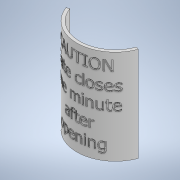
# Autodesk Inventor part: warningSign
Saved by Autodesk Inventor 2021.2 (Build 252289000, 289)
## iProperties
Created: 2020-11-24
Part Number: warningSign
Material: Generic
Document SubType Name: Modeling
Designer: robst
Density: 1 g/cm^3
Appearance: Default
Author: robst
Autodesk Inventor part; units mm, degrees
(part 1 of 2)
ref_plane "YZ Plane" through (0, 0, 0) normal (1, 0, 0) x (0, 1, 0)
ref_plane "XZ Plane" through (0, 0, 0) normal (0, 1, 0) x (-1, 0, 0)
sketch "Sketch1" plane through (0, 0, 0) normal (0, 1, 0) x (-1, 0, 0)
  arc A0 (65.9911, 38.1) -> (-65.4234, 39.0668) centre (0, 0) ccw
  arc A1 (72.6124, 39.2675) -> (-71.4904, 41.275) centre (0, 0) ccw
  line L0 (0, 0) -> (0, -82.55) construction
  arc A2 (71.6046, 26.0619) -> (-71.6046, 26.0619) centre (0, 0) ccw
  arc A3 (77.5716, 28.2338) -> (-77.5716, 28.2338) centre (0, 0) ccw
  line L1 (0, 0) -> (77.5716, 28.2338) construction
  line L2 (0, 0) -> (-77.5716, 28.2338) construction
  line L3 (-77.5716, 28.2338) -> (-71.6046, 26.0619)
  line L4 (77.5716, 28.2338) -> (71.6046, 26.0619)
  point P0 (-65.4234, 39.0668)
  point P1 (65.9911, 38.1)
  point P2 (72.6124, 39.2675)
  point P3 (-71.4904, 41.275)
  dimension "d0" = 152.4
  dimension "d9" = 6.35
  dimension "d10" = 110
  dimension "d11" = 110
  constraints: 10 end point, 8 point on circle, 4 centre point, 4 coincident, 2 concentric, 2 point on line, 1 vertical
  measures "d0" diameter of A0
  measures "d9" radial gap between concentric circles of A1 A0
  measures "d10" angle of L1 L0
  measures "d11" angle of L2 L0
extrude "Extrusion1" add sketch "Sketch1" along normal blind 203.2
ref_plane "Work Plane1" through (0, 0, 82.55) normal (0, 0, 1) x (1, 0, 0)
sketch "Sketch3" plane through (0, 0, 82.55) normal (0, 0, 1) x (1, 0, 0)
  line L0 (-72.043, 0) -> (-72.043, 203.2) projected
  line L1 (71.4904, 0) -> (71.4904, 203.2) projected
  line L2 (77.5716, 203.2) -> (-77.5716, 203.2) projected
  line L3 (77.5716, 0) -> (-77.5716, 0) projected
  line L4 (-72.043, 177.8) -> (71.4904, 177.8) construction
  spline S0 degree 2 poles (-53.3534, 166.2913) (-55.5146, 166.2913) (-59.1708, 167.7501) (-60.5035, 169.209) knots 0 0 0 1 2 2 2
  spline S1 degree 2 poles (-60.5035, 169.209) (-61.8363, 170.6498) (-63.2952, 174.9723) (-63.2952, 177.782) knots 0 0 0 1 2 2 2
  spline S2 degree 2 poles (-63.2952, 177.782) (-63.2952, 180.5736) (-61.8723, 184.716) (-60.5215, 186.2469) knots 0 0 0 1 2 2 2
  spline S3 degree 2 poles (-60.5215, 186.2469) (-59.1888, 187.7418) (-55.5506, 189.3087) (-53.2993, 189.3087) knots 0 0 0 1 2 2 2
  spline S4 degree 2 poles (-53.2993, 189.3087) (-52.1827, 189.3087) (-50.2195, 188.9845) (-49.391, 188.7324) knots 0 0 0 1 2 2 2
  spline S5 degree 2 poles (-49.391, 188.7324) (-48.6706, 188.4983) (-47.1757, 187.8319) (-46.4373, 187.4356) knots 0 0 0 1 2 2 2
  line L5 (-46.4373, 187.4356) -> (-46.4373, 183.8696)
  line L6 (-46.4373, 183.8696) -> (-46.6714, 183.8696)
  spline S6 degree 2 poles (-46.6714, 183.8696) (-47.0677, 184.2298) (-48.2924, 185.2384) (-49.1749, 185.7246) knots 0 0 0 1 2 2 2
  spline S7 degree 2 poles (-49.1749, 185.7246) (-50.0214, 186.1929) (-52.0206, 186.7873) (-53.3173, 186.7873) knots 0 0 0 1 2 2 2
  spline S8 degree 2 poles (-53.3173, 186.7873) (-54.7402, 186.7873) (-57.2796, 185.6166) (-58.2342, 184.4999) knots 0 0 0 1 2 2 2
  spline S9 degree 2 poles (-58.2342, 184.4999) (-59.1708, 183.3653) (-60.2154, 179.9252) (-60.2154, 177.782) knots 0 0 0 1 2 2 2
  spline S10 degree 2 poles (-60.2154, 177.782) (-60.2154, 175.4947) (-59.1167, 172.1987) (-58.1622, 171.0641) knots 0 0 0 1 2 2 2
  spline S11 degree 2 poles (-58.1622, 171.0641) (-57.2256, 169.9654) (-54.7222, 168.8488) (-53.3173, 168.8488) knots 0 0 0 1 2 2 2
  spline S12 degree 2 poles (-53.3173, 168.8488) (-52.0386, 168.8488) (-49.8593, 169.4791) (-49.0128, 169.9474) knots 0 0 0 1 2 2 2
  spline S13 degree 2 poles (-49.0128, 169.9474) (-48.2023, 170.4157) (-46.9956, 171.3882) (-46.6534, 171.7304) knots 0 0 0 1 2 2 2
  line L7 (-46.6534, 171.7304) -> (-46.4373, 171.7304)
  line L8 (-46.4373, 171.7304) -> (-46.4373, 168.2004)
  spline S14 degree 2 poles (-46.4373, 168.2004) (-47.1757, 167.8582) (-48.4725, 167.2278) (-49.391, 166.9396) knots 0 0 0 1 2 2 2
  spline S15 degree 2 poles (-49.391, 166.9396) (-50.3636, 166.6155) (-52.0206, 166.2913) (-53.3534, 166.2913) knots 0 0 0 1 2 2 2
  line L9 (-46.0771, 166.6875) -> (-38.5847, 188.9125)
  line L10 (-38.5847, 188.9125) -> (-34.9466, 188.9125)
  line L11 (-34.9466, 188.9125) -> (-27.4542, 166.6875)
  line L12 (-27.4542, 166.6875) -> (-30.57, 166.6875)
  line L13 (-30.57, 166.6875) -> (-32.5872, 172.9011)
  line L14 (-32.5872, 172.9011) -> (-41.0702, 172.9011)
  line L15 (-41.0702, 172.9011) -> (-43.0873, 166.6875)
  line L16 (-43.0873, 166.6875) -> (-46.0771, 166.6875)
  line L17 (-33.3977, 175.4226) -> (-36.8377, 185.8867)
  line L18 (-36.8377, 185.8867) -> (-40.2597, 175.4226)
  line L19 (-40.2597, 175.4226) -> (-33.3977, 175.4226)
  spline S16 degree 2 poles (-17.2963, 166.2192) (-19.2594, 166.2192) (-22.1771, 167.2458) (-23.2037, 168.2724) knots 0 0 0 1 2 2 2
  spline S17 degree 2 poles (-23.2037, 168.2724) (-24.3744, 169.4251) (-25.329, 172.667) (-25.329, 175.0444) knots 0 0 0 1 2 2 2
  line L20 (-25.329, 175.0444) -> (-25.329, 188.9125)
  line L21 (-25.329, 188.9125) -> (-22.3752, 188.9125)
  line L22 (-22.3752, 188.9125) -> (-22.3752, 175.0444)
  spline S18 degree 2 poles (-22.3752, 175.0444) (-22.3752, 173.4955) (-21.979, 171.4063) (-21.4207, 170.5598) knots 0 0 0 1 2 2 2
  spline S19 degree 2 poles (-21.4207, 170.5598) (-20.8263, 169.6592) (-18.7731, 168.7407) (-17.2963, 168.7407) knots 0 0 0 1 2 2 2
  spline S20 degree 2 poles (-17.2963, 168.7407) (-15.9094, 168.7407) (-13.7482, 169.6592) (-13.1538, 170.5598) knots 0 0 0 1 2 2 2
  spline S21 degree 2 poles (-13.1538, 170.5598) (-12.5955, 171.4063) (-12.1993, 173.4775) (-12.1993, 174.9723) knots 0 0 0 1 2 2 2
  line L23 (-12.1993, 174.9723) -> (-12.1993, 188.9125)
  line L24 (-12.1993, 188.9125) -> (-9.2456, 188.9125)
  line L25 (-9.2456, 188.9125) -> (-9.2456, 175.0444)
  spline S22 degree 2 poles (-9.2456, 175.0444) (-9.2456, 172.721) (-10.1821, 169.4071) (-11.3708, 168.2724) knots 0 0 0 1 2 2 2
  spline S23 degree 2 poles (-11.3708, 168.2724) (-12.4334, 167.2278) (-15.2431, 166.2192) (-17.2963, 166.2192) knots 0 0 0 1 2 2 2
  line L26 (0.174, 166.6875) -> (0.174, 186.283)
  line L27 (0.174, 186.283) -> (-7.2824, 186.283)
  line L28 (-7.2824, 186.283) -> (-7.2824, 188.9125)
  line L29 (-7.2824, 188.9125) -> (10.584, 188.9125)
  line L30 (10.584, 188.9125) -> (10.584, 186.283)
  line L31 (10.584, 186.283) -> (3.1277, 186.283)
  line L32 (3.1277, 186.283) -> (3.1277, 166.6875)
  line L33 (3.1277, 166.6875) -> (0.174, 166.6875)
  line L34 (20.5979, 166.6875) -> (11.9889, 166.6875)
  line L35 (11.9889, 166.6875) -> (11.9889, 168.9568)
  line L36 (11.9889, 168.9568) -> (14.8165, 168.9568)
  line L37 (14.8165, 168.9568) -> (14.8165, 186.6432)
  line L38 (14.8165, 186.6432) -> (11.9889, 186.6432)
  line L39 (11.9889, 186.6432) -> (11.9889, 188.9125)
  line L40 (11.9889, 188.9125) -> (20.5979, 188.9125)
  line L41 (20.5979, 188.9125) -> (20.5979, 186.6432)
  line L42 (20.5979, 186.6432) -> (17.7703, 186.6432)
  line L43 (17.7703, 186.6432) -> (17.7703, 168.9568)
  line L44 (17.7703, 168.9568) -> (20.5979, 168.9568)
  line L45 (20.5979, 168.9568) -> (20.5979, 166.6875)
  spline S24 degree 2 poles (39.9772, 186.373) (41.238, 184.8962) (42.6428, 180.5736) (42.6428, 177.8) knots 0 0 0 1 2 2 2
  spline S25 degree 2 poles (42.6428, 177.8) (42.6428, 175.0984) (41.274, 170.7219) (39.9772, 169.245) knots 0 0 0 1 2 2 2
  spline S26 degree 2 poles (39.9772, 169.245) (38.6084, 167.6961) (34.9883, 166.2192) (32.809, 166.2192) knots 0 0 0 1 2 2 2
  spline S27 degree 2 poles (32.809, 166.2192) (30.5577, 166.2192) (26.9556, 167.7501) (25.6409, 169.245) knots 0 0 0 1 2 2 2
  spline S28 degree 2 poles (25.6409, 169.245) (24.3621, 170.7219) (22.9933, 175.0624) (22.9933, 177.8) knots 0 0 0 1 2 2 2
  spline S29 degree 2 poles (22.9933, 177.8) (22.9933, 180.5916) (24.3801, 184.8421) (25.6589, 186.373) knots 0 0 0 1 2 2 2
  spline S30 degree 2 poles (25.6589, 186.373) (26.9556, 187.8499) (30.5757, 189.3808) (32.809, 189.3808) knots 0 0 0 1 2 2 2
  spline S31 degree 2 poles (32.809, 189.3808) (35.0784, 189.3808) (38.7165, 187.7958) (39.9772, 186.373) knots 0 0 0 1 2 2 2
  spline S32 degree 2 poles (39.563, 177.8) (39.563, 179.9973) (38.6084, 183.4013) (37.7439, 184.5179) knots 0 0 0 1 2 2 2
  spline S33 degree 2 poles (37.7439, 184.5179) (36.8614, 185.6706) (34.376, 186.8233) (32.8271, 186.8233) knots 0 0 0 1 2 2 2
  spline S34 degree 2 poles (32.8271, 186.8233) (31.2241, 186.8233) (28.8107, 185.7066) (27.8922, 184.5179) knots 0 0 0 1 2 2 2
  spline S35 degree 2 poles (27.8922, 184.5179) (27.0097, 183.3833) (26.0731, 179.9613) (26.0731, 177.8) knots 0 0 0 1 2 2 2
  spline S36 degree 2 poles (26.0731, 177.8) (26.0731, 173.4234) (29.7473, 168.7767) (32.8271, 168.7767) knots 0 0 0 1 2 2 2
  spline S37 degree 2 poles (32.8271, 168.7767) (35.9069, 168.7767) (39.563, 173.4234) (39.563, 177.8) knots 0 0 0 1 2 2 2
  line L46 (61.788, 166.6875) -> (58.4741, 166.6875)
  line L47 (58.4741, 166.6875) -> (48.6403, 185.8507)
  line L48 (48.6403, 185.8507) -> (48.6403, 166.6875)
  line L49 (48.6403, 166.6875) -> (45.8847, 166.6875)
  line L50 (45.8847, 166.6875) -> (45.8847, 188.9125)
  line L51 (45.8847, 188.9125) -> (50.0812, 188.9125)
  line L52 (50.0812, 188.9125) -> (59.0324, 171.3162)
  line L53 (59.0324, 171.3162) -> (59.0324, 188.9125)
  line L54 (59.0324, 188.9125) -> (61.788, 188.9125)
  line L55 (61.788, 188.9125) -> (61.788, 166.6875)
  spline S38 degree 2 poles (-65.3844, 129.0315) (-67.7438, 129.0315) (-71.6521, 130.4723) (-73.0569, 131.9312) knots 0 0 0 1 2 2 2
  spline S39 degree 2 poles (-73.0569, 131.9312) (-74.4617, 133.408) (-75.9566, 137.7666) (-75.9566, 140.5942) knots 0 0 0 1 2 2 2
  spline S40 degree 2 poles (-75.9566, 140.5942) (-75.9566, 143.2778) (-74.4437, 147.5283) (-73.0389, 149.0412) knots 0 0 0 1 2 2 2
  spline S41 degree 2 poles (-73.0389, 149.0412) (-71.6881, 150.5) (-67.7258, 152.085) (-65.3664, 152.085) knots 0 0 0 1 2 2 2
  spline S42 degree 2 poles (-65.3664, 152.085) (-64.2317, 152.085) (-62.1785, 151.7608) (-61.242, 151.4726) knots 0 0 0 1 2 2 2
  spline S43 degree 2 poles (-61.242, 151.4726) (-60.4855, 151.2565) (-58.6484, 150.464) (-58.0901, 150.1759) knots 0 0 0 1 2 2 2
  line L56 (-58.0901, 150.1759) -> (-58.0901, 146.6098)
  line L57 (-58.0901, 146.6098) -> (-58.3423, 146.6098)
  spline S44 degree 2 poles (-58.3423, 146.6098) (-58.9006, 147.096) (-60.0713, 147.9786) (-61.1519, 148.4829) knots 0 0 0 1 2 2 2
  spline S45 degree 2 poles (-61.1519, 148.4829) (-62.0524, 148.9331) (-64.3758, 149.5275) (-65.7086, 149.5275) knots 0 0 0 1 2 2 2
  spline S46 degree 2 poles (-65.7086, 149.5275) (-68.9145, 149.5275) (-72.8768, 144.7006) (-72.8768, 140.6843) knots 0 0 0 1 2 2 2
  spline S47 degree 2 poles (-72.8768, 140.6843) (-72.8768, 138.451) (-71.8322, 135.101) (-70.8416, 133.9484) knots 0 0 0 1 2 2 2
  spline S48 degree 2 poles (-70.8416, 133.9484) (-69.887, 132.7957) (-67.1854, 131.589) (-65.4925, 131.589) knots 0 0 0 1 2 2 2
  spline S49 degree 2 poles (-65.4925, 131.589) (-64.2497, 131.589) (-61.7643, 131.9492) (-60.9178, 132.3094) knots 0 0 0 1 2 2 2
  line L58 (-60.9178, 132.3094) -> (-60.9178, 138.0548)
  line L59 (-60.9178, 138.0548) -> (-66.0688, 138.0548)
  line L60 (-66.0688, 138.0548) -> (-66.0688, 140.6483)
  line L61 (-66.0688, 140.6483) -> (-58.0001, 140.6483)
  line L62 (-58.0001, 140.6483) -> (-58.0001, 130.9406)
  spline S50 degree 2 poles (-58.0001, 130.9406) (-58.5584, 130.6885) (-60.4675, 129.914) (-61.278, 129.6799) knots 0 0 0 1 2 2 2
  spline S51 degree 2 poles (-61.278, 129.6799) (-62.3766, 129.3557) (-64.1417, 129.0315) (-65.3844, 129.0315) knots 0 0 0 1 2 2 2
  spline S52 degree 2 poles (-45.2126, 131.2288) (-45.5548, 130.9766) (-46.7075, 130.0761) (-47.2478, 129.8059) knots 0 0 0 1 2 2 2
  spline S53 degree 2 poles (-47.2478, 129.8059) (-47.9862, 129.4097) (-49.373, 128.9955) (-50.6338, 128.9955) knots 0 0 0 1 2 2 2
  spline S54 degree 2 poles (-50.6338, 128.9955) (-51.6604, 128.9955) (-53.5154, 129.7699) (-54.2179, 130.4723) knots 0 0 0 1 2 2 2
  spline S55 degree 2 poles (-54.2179, 130.4723) (-54.8842, 131.1567) (-55.6947, 133.1739) (-55.6947, 134.2906) knots 0 0 0 1 2 2 2
  spline S56 degree 2 poles (-55.6947, 134.2906) (-55.6947, 136.0196) (-54.2359, 138.469) (-52.6509, 139.1714) knots 0 0 0 1 2 2 2
  spline S57 degree 2 poles (-52.6509, 139.1714) (-51.2461, 139.8198) (-47.4279, 140.3061) (-45.2126, 140.4322) knots 0 0 0 1 2 2 2
  line L63 (-45.2126, 140.4322) -> (-45.2126, 140.9725)
  spline S58 degree 2 poles (-45.2126, 140.9725) (-45.2126, 141.945) (-45.8069, 143.1517) (-46.3473, 143.4939) knots 0 0 0 1 2 2 2
  spline S59 degree 2 poles (-46.3473, 143.4939) (-46.8876, 143.8361) (-48.4365, 144.0523) (-49.265, 144.0523) knots 0 0 0 1 2 2 2
  spline S60 degree 2 poles (-49.265, 144.0523) (-50.2375, 144.0523) (-52.8671, 143.4759) (-54.1818, 142.9176) knots 0 0 0 1 2 2 2
  line L64 (-54.1818, 142.9176) -> (-54.3439, 142.9176)
  line L65 (-54.3439, 142.9176) -> (-54.3439, 145.7813)
  spline S61 degree 2 poles (-54.3439, 145.7813) (-53.5695, 145.9974) (-50.6698, 146.5377) (-49.2469, 146.5377) knots 0 0 0 1 2 2 2
  spline S62 degree 2 poles (-49.2469, 146.5377) (-47.5179, 146.5377) (-45.1586, 145.9974) (-44.222, 145.295) knots 0 0 0 1 2 2 2
  spline S63 degree 2 poles (-44.222, 145.295) (-43.3035, 144.6106) (-42.4029, 142.4313) (-42.4029, 140.8644) knots 0 0 0 1 2 2 2
  line L66 (-42.4029, 140.8644) -> (-42.4029, 129.4637)
  line L67 (-42.4029, 129.4637) -> (-45.2126, 129.4637)
  line L68 (-45.2126, 129.4637) -> (-45.2126, 131.2288)
  line L69 (-45.2126, 133.5701) -> (-45.2126, 138.1988)
  spline S64 degree 2 poles (-45.2126, 138.1988) (-46.2212, 138.1088) (-49.265, 137.8026) (-50.2195, 137.5144) knots 0 0 0 1 2 2 2
  spline S65 degree 2 poles (-50.2195, 137.5144) (-51.3362, 137.1722) (-52.795, 135.7494) (-52.795, 134.4887) knots 0 0 0 1 2 2 2
  spline S66 degree 2 poles (-52.795, 134.4887) (-52.795, 133.0478) (-51.1741, 131.589) (-49.6252, 131.589) knots 0 0 0 1 2 2 2
  spline S67 degree 2 poles (-49.6252, 131.589) (-48.3104, 131.589) (-46.1491, 132.7236) (-45.2126, 133.5701) knots 0 0 0 1 2 2 2
  spline S68 degree 2 poles (-33.4157, 129.1395) (-35.703, 129.1395) (-38.2785, 131.7511) (-38.2785, 134.5787) knots 0 0 0 1 2 2 2
  line L70 (-38.2785, 134.5787) -> (-38.2785, 143.8181)
  line L71 (-38.2785, 143.8181) -> (-40.1696, 143.8181)
  line L72 (-40.1696, 143.8181) -> (-40.1696, 146.1415)
  line L73 (-40.1696, 146.1415) -> (-38.2785, 146.1415)
  line L74 (-38.2785, 146.1415) -> (-38.2785, 150.9323)
  line L75 (-38.2785, 150.9323) -> (-35.4689, 150.9323)
  line L76 (-35.4689, 150.9323) -> (-35.4689, 146.1415)
  line L77 (-35.4689, 146.1415) -> (-30.2999, 146.1415)
  line L78 (-30.2999, 146.1415) -> (-30.2999, 143.8181)
  line L79 (-30.2999, 143.8181) -> (-35.4689, 143.8181)
  line L80 (-35.4689, 143.8181) -> (-35.4689, 135.8755)
  spline S69 degree 2 poles (-35.4689, 135.8755) (-35.4689, 134.6147) (-35.3788, 133.2279) (-35.0727, 132.6336) knots 0 0 0 1 2 2 2
  spline S70 degree 2 poles (-35.0727, 132.6336) (-34.8205, 132.1113) (-33.6858, 131.589) (-32.7133, 131.589) knots 0 0 0 1 2 2 2
  spline S71 degree 2 poles (-32.7133, 131.589) (-32.0289, 131.589) (-30.7501, 132.0032) (-30.462, 132.1293) knots 0 0 0 1 2 2 2
  line L81 (-30.462, 132.1293) -> (-30.2999, 132.1293)
  line L82 (-30.2999, 132.1293) -> (-30.2999, 129.6078)
  spline S72 degree 2 poles (-30.2999, 129.6078) (-31.0923, 129.3917) (-32.7133, 129.1395) (-33.4157, 129.1395) knots 0 0 0 1 2 2 2
  spline S73 degree 2 poles (-20.9884, 129.0855) (-24.9868, 129.0855) (-29.3813, 133.5701) (-29.3813, 137.7126) knots 0 0 0 1 2 2 2
  spline S74 degree 2 poles (-29.3813, 137.7126) (-29.3813, 141.7829) (-25.1128, 146.6098) (-21.6728, 146.6098) knots 0 0 0 1 2 2 2
  spline S75 degree 2 poles (-21.6728, 146.6098) (-20.1239, 146.6098) (-17.7285, 145.7092) (-16.846, 144.7547) knots 0 0 0 1 2 2 2
  spline S76 degree 2 poles (-16.846, 144.7547) (-15.9455, 143.8001) (-14.9909, 141.0445) (-14.9909, 139.0453) knots 0 0 0 1 2 2 2
  line L83 (-14.9909, 139.0453) -> (-14.9909, 137.5144)
  line L84 (-14.9909, 137.5144) -> (-26.5357, 137.5144)
  spline S77 degree 2 poles (-26.5357, 137.5144) (-26.5357, 134.6147) (-23.618, 131.5349) (-21.0244, 131.5349) knots 0 0 0 1 2 2 2
  spline S78 degree 2 poles (-21.0244, 131.5349) (-20.1059, 131.5349) (-18.3229, 131.9492) (-17.6024, 132.2734) knots 0 0 0 1 2 2 2
  spline S79 degree 2 poles (-17.6024, 132.2734) (-16.846, 132.6336) (-15.8014, 133.264) (-15.4592, 133.5521) knots 0 0 0 1 2 2 2
  line L85 (-15.4592, 133.5521) -> (-15.2971, 133.5521)
  line L86 (-15.2971, 133.5521) -> (-15.2971, 130.4903)
  spline S80 degree 2 poles (-15.2971, 130.4903) (-15.7834, 130.2922) (-17.2602, 129.7159) (-17.8366, 129.5538) knots 0 0 0 1 2 2 2
  spline S81 degree 2 poles (-17.8366, 129.5538) (-18.647, 129.3196) (-19.9798, 129.0855) (-20.9884, 129.0855) knots 0 0 0 1 2 2 2
  spline S82 degree 2 poles (-17.7285, 139.6577) (-17.7645, 140.7924) (-18.2328, 142.4493) (-18.6831, 143.0077) knots 0 0 0 1 2 2 2
  spline S83 degree 2 poles (-18.6831, 143.0077) (-19.1694, 143.638) (-20.7002, 144.3044) (-21.8349, 144.3044) knots 0 0 0 1 2 2 2
  spline S84 degree 2 poles (-21.8349, 144.3044) (-22.9516, 144.3044) (-24.5185, 143.638) (-25.1669, 142.9896) knots 0 0 0 1 2 2 2
  spline S85 degree 2 poles (-25.1669, 142.9896) (-25.7972, 142.3233) (-26.4456, 140.7203) (-26.5357, 139.6577) knots 0 0 0 1 2 2 2
  line L87 (-26.5357, 139.6577) -> (-17.7285, 139.6577)
  spline S86 degree 2 poles (4.0282, 129.0855) (2.2992, 129.0855) (-0.5645, 130.1481) (-1.5911, 131.2288) knots 0 0 0 1 2 2 2
  spline S87 degree 2 poles (-1.5911, 131.2288) (-2.6177, 132.2914) (-3.7523, 135.5693) (-3.7523, 137.7666) knots 0 0 0 1 2 2 2
  spline S88 degree 2 poles (-3.7523, 137.7666) (-3.7523, 139.9639) (-2.5817, 143.1698) (-1.5911, 144.2504) knots 0 0 0 1 2 2 2
  spline S89 degree 2 poles (-1.5911, 144.2504) (-0.6005, 145.349) (2.3352, 146.5197) (4.0282, 146.5197) knots 0 0 0 1 2 2 2
  spline S90 degree 2 poles (4.0282, 146.5197) (5.397, 146.5197) (7.9545, 145.7453) (8.9451, 145.241) knots 0 0 0 1 2 2 2
  line L88 (8.9451, 145.241) -> (8.9451, 142.0891)
  line L89 (8.9451, 142.0891) -> (8.783, 142.0891)
  spline S91 degree 2 poles (8.783, 142.0891) (8.4768, 142.3413) (7.5403, 142.9896) (6.8739, 143.3318) knots 0 0 0 1 2 2 2
  spline S92 degree 2 poles (6.8739, 143.3318) (6.2795, 143.62) (4.6946, 144.0703) (3.9742, 144.0703) knots 0 0 0 1 2 2 2
  spline S93 degree 2 poles (3.9742, 144.0703) (1.7949, 144.0703) (-0.8526, 140.7744) (-0.8526, 137.7666) knots 0 0 0 1 2 2 2
  spline S94 degree 2 poles (-0.8526, 137.7666) (-0.8526, 134.8309) (1.7049, 131.5349) (3.9742, 131.5349) knots 0 0 0 1 2 2 2
  spline S95 degree 2 poles (3.9742, 131.5349) (5.343, 131.5349) (7.8284, 132.6696) (8.783, 133.5521) knots 0 0 0 1 2 2 2
  line L90 (8.783, 133.5521) -> (8.9451, 133.5521)
  line L91 (8.9451, 133.5521) -> (8.9451, 130.4003)
  spline S96 degree 2 poles (8.9451, 130.4003) (8.5308, 130.2022) (7.2701, 129.6438) (6.7658, 129.5178) knots 0 0 0 1 2 2 2
  spline S97 degree 2 poles (6.7658, 129.5178) (6.0454, 129.3016) (4.9107, 129.0855) (4.0282, 129.0855) knots 0 0 0 1 2 2 2
  line L92 (14.3663, 129.4637) -> (11.5566, 129.4637)
  line L93 (11.5566, 129.4637) -> (11.5566, 152.6793)
  line L94 (11.5566, 152.6793) -> (14.3663, 152.6793)
  line L95 (14.3663, 152.6793) -> (14.3663, 129.4637)
  spline S98 degree 2 poles (32.1967, 137.8026) (32.1967, 133.5881) (28.1443, 128.9955) (24.7583, 128.9955) knots 0 0 0 1 2 2 2
  spline S99 degree 2 poles (24.7583, 128.9955) (21.2823, 128.9955) (17.302, 133.7322) (17.302, 137.8026) knots 0 0 0 1 2 2 2
  spline S100 degree 2 poles (17.302, 137.8026) (17.302, 141.9811) (21.4084, 146.6098) (24.7583, 146.6098) knots 0 0 0 1 2 2 2
  spline S101 degree 2 poles (24.7583, 146.6098) (28.1443, 146.6098) (32.1967, 141.9991) (32.1967, 137.8026) knots 0 0 0 1 2 2 2
  spline S102 degree 2 poles (29.297, 137.8026) (29.297, 141.0445) (26.9376, 144.1964) (24.7583, 144.1964) knots 0 0 0 1 2 2 2
  spline S103 degree 2 poles (24.7583, 144.1964) (22.5791, 144.1964) (20.2017, 141.0445) (20.2017, 137.8026) knots 0 0 0 1 2 2 2
  spline S104 degree 2 poles (20.2017, 137.8026) (20.2017, 134.6508) (22.5791, 131.4089) (24.7583, 131.4089) knots 0 0 0 1 2 2 2
  spline S105 degree 2 poles (24.7583, 131.4089) (26.9196, 131.4089) (29.297, 134.5967) (29.297, 137.8026) knots 0 0 0 1 2 2 2
  spline S106 degree 2 poles (39.581, 129.0675) (37.906, 129.0675) (35.0063, 129.968) (34.0518, 130.4723) knots 0 0 0 1 2 2 2
  line L96 (34.0518, 130.4723) -> (34.0518, 133.6242)
  line L97 (34.0518, 133.6242) -> (34.1959, 133.6242)
  spline S107 degree 2 poles (34.1959, 133.6242) (34.5561, 133.336) (35.5286, 132.6516) (36.3391, 132.2734) knots 0 0 0 1 2 2 2
  spline S108 degree 2 poles (36.3391, 132.2734) (37.0415, 131.9312) (38.7705, 131.4269) (39.6891, 131.4269) knots 0 0 0 1 2 2 2
  spline S109 degree 2 poles (39.6891, 131.4269) (40.3555, 131.4269) (41.8864, 131.7331) (42.2466, 131.9852) knots 0 0 0 1 2 2 2
  spline S110 degree 2 poles (42.2466, 131.9852) (42.7689, 132.3274) (43.2372, 133.1019) (43.2372, 133.8943) knots 0 0 0 1 2 2 2
  spline S111 degree 2 poles (43.2372, 133.8943) (43.2372, 134.8849) (42.1565, 135.9115) (40.7697, 136.2537) knots 0 0 0 1 2 2 2
  spline S112 degree 2 poles (40.7697, 136.2537) (40.2294, 136.3798) (38.5004, 136.74) (37.7619, 136.9381) knots 0 0 0 1 2 2 2
  spline S113 degree 2 poles (37.7619, 136.9381) (35.8528, 137.4964) (34.1238, 139.8018) (34.1238, 141.4407) knots 0 0 0 1 2 2 2
  spline S114 degree 2 poles (34.1238, 141.4407) (34.1238, 143.7101) (37.5278, 146.5377) (40.3375, 146.5377) knots 0 0 0 1 2 2 2
  spline S115 degree 2 poles (40.3375, 146.5377) (41.7243, 146.5377) (44.5339, 145.8533) (45.4885, 145.331) knots 0 0 0 1 2 2 2
  line L98 (45.4885, 145.331) -> (45.4885, 142.3233)
  line L99 (45.4885, 142.3233) -> (45.3444, 142.3233)
  spline S116 degree 2 poles (45.3444, 142.3233) (44.2638, 143.1878) (41.6342, 144.1783) (40.2834, 144.1783) knots 0 0 0 1 2 2 2
  spline S117 degree 2 poles (40.2834, 144.1783) (38.8966, 144.1783) (36.9875, 143.0077) (36.9875, 141.837) knots 0 0 0 1 2 2 2
  spline S118 degree 2 poles (36.9875, 141.837) (36.9875, 140.7744) (38.1222, 139.7477) (39.3829, 139.4236) knots 0 0 0 1 2 2 2
  spline S119 degree 2 poles (39.3829, 139.4236) (39.9953, 139.2615) (41.5442, 138.9373) (42.3907, 138.7392) knots 0 0 0 1 2 2 2
  spline S120 degree 2 poles (42.3907, 138.7392) (44.2277, 138.2709) (46.1008, 136.1276) (46.1008, 134.2725) knots 0 0 0 1 2 2 2
  spline S121 degree 2 poles (46.1008, 134.2725) (46.1008, 133.1919) (45.2543, 131.2828) (44.4258, 130.5804) knots 0 0 0 1 2 2 2
  spline S122 degree 2 poles (44.4258, 130.5804) (43.5433, 129.842) (41.292, 129.0675) (39.581, 129.0675) knots 0 0 0 1 2 2 2
  spline S123 degree 2 poles (55.9526, 129.0855) (51.9543, 129.0855) (47.5597, 133.5701) (47.5597, 137.7126) knots 0 0 0 1 2 2 2
  spline S124 degree 2 poles (47.5597, 137.7126) (47.5597, 141.7829) (51.8282, 146.6098) (55.2682, 146.6098) knots 0 0 0 1 2 2 2
  spline S125 degree 2 poles (55.2682, 146.6098) (56.8171, 146.6098) (59.2125, 145.7092) (60.095, 144.7547) knots 0 0 0 1 2 2 2
  spline S126 degree 2 poles (60.095, 144.7547) (60.9955, 143.8001) (61.9501, 141.0445) (61.9501, 139.0453) knots 0 0 0 1 2 2 2
  line L100 (61.9501, 139.0453) -> (61.9501, 137.5144)
  line L101 (61.9501, 137.5144) -> (50.4053, 137.5144)
  spline S127 degree 2 poles (50.4053, 137.5144) (50.4053, 134.6147) (53.3231, 131.5349) (55.9166, 131.5349) knots 0 0 0 1 2 2 2
  spline S128 degree 2 poles (55.9166, 131.5349) (56.8351, 131.5349) (58.6181, 131.9492) (59.3386, 132.2734) knots 0 0 0 1 2 2 2
  spline S129 degree 2 poles (59.3386, 132.2734) (60.095, 132.6336) (61.1396, 133.264) (61.4818, 133.5521) knots 0 0 0 1 2 2 2
  line L102 (61.4818, 133.5521) -> (61.6439, 133.5521)
  line L103 (61.6439, 133.5521) -> (61.6439, 130.4903)
  spline S130 degree 2 poles (61.6439, 130.4903) (61.1576, 130.2922) (59.6808, 129.7159) (59.1044, 129.5538) knots 0 0 0 1 2 2 2
  spline S131 degree 2 poles (59.1044, 129.5538) (58.294, 129.3196) (56.9612, 129.0855) (55.9526, 129.0855) knots 0 0 0 1 2 2 2
  spline S132 degree 2 poles (59.2125, 139.6577) (59.1765, 140.7924) (58.7082, 142.4493) (58.2579, 143.0077) knots 0 0 0 1 2 2 2
  spline S133 degree 2 poles (58.2579, 143.0077) (57.7717, 143.638) (56.2408, 144.3044) (55.1061, 144.3044) knots 0 0 0 1 2 2 2
  spline S134 degree 2 poles (55.1061, 144.3044) (53.9894, 144.3044) (52.4225, 143.638) (51.7741, 142.9896) knots 0 0 0 1 2 2 2
  spline S135 degree 2 poles (51.7741, 142.9896) (51.1438, 142.3233) (50.4954, 140.7203) (50.4053, 139.6577) knots 0 0 0 1 2 2 2
  line L104 (50.4053, 139.6577) -> (59.2125, 139.6577)
  spline S136 degree 2 poles (69.2984, 129.0675) (67.6234, 129.0675) (64.7237, 129.968) (63.7692, 130.4723) knots 0 0 0 1 2 2 2
  line L105 (63.7692, 130.4723) -> (63.7692, 133.6242)
  line L106 (63.7692, 133.6242) -> (63.9132, 133.6242)
  spline S137 degree 2 poles (63.9132, 133.6242) (64.2735, 133.336) (65.246, 132.6516) (66.0565, 132.2734) knots 0 0 0 1 2 2 2
  spline S138 degree 2 poles (66.0565, 132.2734) (66.7589, 131.9312) (68.4879, 131.4269) (69.4065, 131.4269) knots 0 0 0 1 2 2 2
  spline S139 degree 2 poles (69.4065, 131.4269) (70.0728, 131.4269) (71.6037, 131.7331) (71.964, 131.9852) knots 0 0 0 1 2 2 2
  spline S140 degree 2 poles (71.964, 131.9852) (72.4863, 132.3274) (72.9545, 133.1019) (72.9545, 133.8943) knots 0 0 0 1 2 2 2
  spline S141 degree 2 poles (72.9545, 133.8943) (72.9545, 134.8849) (71.8739, 135.9115) (70.4871, 136.2537) knots 0 0 0 1 2 2 2
  spline S142 degree 2 poles (70.4871, 136.2537) (69.9468, 136.3798) (68.2178, 136.74) (67.4793, 136.9381) knots 0 0 0 1 2 2 2
  spline S143 degree 2 poles (67.4793, 136.9381) (65.5702, 137.4964) (63.8412, 139.8018) (63.8412, 141.4407) knots 0 0 0 1 2 2 2
  spline S144 degree 2 poles (63.8412, 141.4407) (63.8412, 143.7101) (67.2452, 146.5377) (70.0548, 146.5377) knots 0 0 0 1 2 2 2
  spline S145 degree 2 poles (70.0548, 146.5377) (71.4417, 146.5377) (74.2513, 145.8533) (75.2059, 145.331) knots 0 0 0 1 2 2 2
  line L107 (75.2059, 145.331) -> (75.2059, 142.3233)
  line L108 (75.2059, 142.3233) -> (75.0618, 142.3233)
  spline S146 degree 2 poles (75.0618, 142.3233) (73.9811, 143.1878) (71.3516, 144.1783) (70.0008, 144.1783) knots 0 0 0 1 2 2 2
  spline S147 degree 2 poles (70.0008, 144.1783) (68.614, 144.1783) (66.7049, 143.0077) (66.7049, 141.837) knots 0 0 0 1 2 2 2
  spline S148 degree 2 poles (66.7049, 141.837) (66.7049, 140.7744) (67.8395, 139.7477) (69.1003, 139.4236) knots 0 0 0 1 2 2 2
  spline S149 degree 2 poles (69.1003, 139.4236) (69.7126, 139.2615) (71.2615, 138.9373) (72.108, 138.7392) knots 0 0 0 1 2 2 2
  spline S150 degree 2 poles (72.108, 138.7392) (73.9451, 138.2709) (75.8182, 136.1276) (75.8182, 134.2725) knots 0 0 0 1 2 2 2
  spline S151 degree 2 poles (75.8182, 134.2725) (75.8182, 133.1919) (74.9717, 131.2828) (74.1432, 130.5804) knots 0 0 0 1 2 2 2
  spline S152 degree 2 poles (74.1432, 130.5804) (73.2607, 129.842) (71.0094, 129.0675) (69.2984, 129.0675) knots 0 0 0 1 2 2 2
  spline S153 degree 2 poles (-60.6836, 101.4253) (-60.6836, 97.2109) (-64.736, 92.6182) (-68.122, 92.6182) knots 0 0 0 1 2 2 2
  spline S154 degree 2 poles (-68.122, 92.6182) (-71.598, 92.6182) (-75.5784, 97.355) (-75.5784, 101.4253) knots 0 0 0 1 2 2 2
  spline S155 degree 2 poles (-75.5784, 101.4253) (-75.5784, 105.6038) (-71.472, 110.2325) (-68.122, 110.2325) knots 0 0 0 1 2 2 2
  spline S156 degree 2 poles (-68.122, 110.2325) (-64.736, 110.2325) (-60.6836, 105.6218) (-60.6836, 101.4253) knots 0 0 0 1 2 2 2
  spline S157 degree 2 poles (-63.5833, 101.4253) (-63.5833, 104.6672) (-65.9427, 107.8191) (-68.122, 107.8191) knots 0 0 0 1 2 2 2
  spline S158 degree 2 poles (-68.122, 107.8191) (-70.3013, 107.8191) (-72.6787, 104.6672) (-72.6787, 101.4253) knots 0 0 0 1 2 2 2
  spline S159 degree 2 poles (-72.6787, 101.4253) (-72.6787, 98.2735) (-70.3013, 95.0316) (-68.122, 95.0316) knots 0 0 0 1 2 2 2
  spline S160 degree 2 poles (-68.122, 95.0316) (-65.9607, 95.0316) (-63.5833, 98.2195) (-63.5833, 101.4253) knots 0 0 0 1 2 2 2
  line L109 (-44.7083, 93.0865) -> (-47.5179, 93.0865)
  line L110 (-47.5179, 93.0865) -> (-47.5179, 102.596)
  spline S161 degree 2 poles (-47.5179, 102.596) (-47.5179, 103.7487) (-47.7341, 105.7299) (-48.0583, 106.3242) knots 0 0 0 1 2 2 2
  spline S162 degree 2 poles (-48.0583, 106.3242) (-48.4005, 106.9546) (-49.6252, 107.5669) (-50.6698, 107.5669) knots 0 0 0 1 2 2 2
  spline S163 degree 2 poles (-50.6698, 107.5669) (-51.7144, 107.5669) (-53.9297, 106.4503) (-54.9923, 105.5498) knots 0 0 0 1 2 2 2
  line L111 (-54.9923, 105.5498) -> (-54.9923, 93.0865)
  line L112 (-54.9923, 93.0865) -> (-57.802, 93.0865)
  line L113 (-57.802, 93.0865) -> (-57.802, 109.7642)
  line L114 (-57.802, 109.7642) -> (-54.9923, 109.7642)
  line L115 (-54.9923, 109.7642) -> (-54.9923, 107.9091)
  spline S164 degree 2 poles (-54.9923, 107.9091) (-53.7316, 109.0438) (-51.3002, 110.2325) (-49.9314, 110.2325) knots 0 0 0 1 2 2 2
  spline S165 degree 2 poles (-49.9314, 110.2325) (-47.4819, 110.2325) (-44.7083, 106.9906) (-44.7083, 103.9108) knots 0 0 0 1 2 2 2
  line L116 (-44.7083, 103.9108) -> (-44.7083, 93.0865)
  spline S166 degree 2 poles (-33.5238, 92.7082) (-37.5221, 92.7082) (-41.9167, 97.1929) (-41.9167, 101.3353) knots 0 0 0 1 2 2 2
  spline S167 degree 2 poles (-41.9167, 101.3353) (-41.9167, 105.4057) (-37.6482, 110.2325) (-34.2082, 110.2325) knots 0 0 0 1 2 2 2
  spline S168 degree 2 poles (-34.2082, 110.2325) (-32.6592, 110.2325) (-30.2638, 109.332) (-29.3813, 108.3774) knots 0 0 0 1 2 2 2
  spline S169 degree 2 poles (-29.3813, 108.3774) (-28.4808, 107.4229) (-27.5262, 104.6672) (-27.5262, 102.6681) knots 0 0 0 1 2 2 2
  line L117 (-27.5262, 102.6681) -> (-27.5262, 101.1372)
  line L118 (-27.5262, 101.1372) -> (-39.071, 101.1372)
  spline S170 degree 2 poles (-39.071, 101.1372) (-39.071, 98.2375) (-36.1533, 95.1577) (-33.5598, 95.1577) knots 0 0 0 1 2 2 2
  spline S171 degree 2 poles (-33.5598, 95.1577) (-32.6412, 95.1577) (-30.8582, 95.5719) (-30.1378, 95.8961) knots 0 0 0 1 2 2 2
  spline S172 degree 2 poles (-30.1378, 95.8961) (-29.3813, 96.2563) (-28.3367, 96.8867) (-27.9945, 97.1749) knots 0 0 0 1 2 2 2
  line L119 (-27.9945, 97.1749) -> (-27.8324, 97.1749)
  line L120 (-27.8324, 97.1749) -> (-27.8324, 94.1131)
  spline S173 degree 2 poles (-27.8324, 94.1131) (-28.3187, 93.9149) (-29.7956, 93.3386) (-30.3719, 93.1765) knots 0 0 0 1 2 2 2
  spline S174 degree 2 poles (-30.3719, 93.1765) (-31.1824, 92.9424) (-32.5152, 92.7082) (-33.5238, 92.7082) knots 0 0 0 1 2 2 2
  spline S175 degree 2 poles (-30.2638, 103.2804) (-30.2999, 104.4151) (-30.7681, 106.0721) (-31.2184, 106.6304) knots 0 0 0 1 2 2 2
  spline S176 degree 2 poles (-31.2184, 106.6304) (-31.7047, 107.2608) (-33.2356, 107.9271) (-34.3702, 107.9271) knots 0 0 0 1 2 2 2
  spline S177 degree 2 poles (-34.3702, 107.9271) (-35.4869, 107.9271) (-37.0538, 107.2608) (-37.7022, 106.6124) knots 0 0 0 1 2 2 2
  spline S178 degree 2 poles (-37.7022, 106.6124) (-38.3326, 105.946) (-38.9809, 104.343) (-39.071, 103.2804) knots 0 0 0 1 2 2 2
  line L121 (-39.071, 103.2804) -> (-30.2638, 103.2804)
  line L122 (3.7761, 93.0865) -> (3.7761, 102.7401)
  spline S179 degree 2 poles (3.7761, 102.7401) (3.7761, 103.8928) (3.596, 105.8559) (3.3078, 106.3962) knots 0 0 0 1 2 2 2
  spline S180 degree 2 poles (3.3078, 106.3962) (3.0196, 106.9906) (1.921, 107.5669) (0.9664, 107.5669) knots 0 0 0 1 2 2 2
  spline S181 degree 2 poles (0.9664, 107.5669) (0.1019, 107.5669) (-1.8792, 106.5043) (-2.9239, 105.4957) knots 0 0 0 1 2 2 2
  spline S182 degree 2 poles (-2.9239, 105.4957) (-2.9058, 105.2436) (-2.8698, 104.5412) (-2.8698, 104.0729) knots 0 0 0 1 2 2 2
  line L123 (-2.8698, 104.0729) -> (-2.8698, 93.0865)
  line L124 (-2.8698, 93.0865) -> (-5.6795, 93.0865)
  line L125 (-5.6795, 93.0865) -> (-5.6795, 102.7401)
  spline S183 degree 2 poles (-5.6795, 102.7401) (-5.6795, 103.8928) (-5.8596, 105.8559) (-6.1477, 106.3962) knots 0 0 0 1 2 2 2
  spline S184 degree 2 poles (-6.1477, 106.3962) (-6.4359, 106.9906) (-7.5345, 107.5669) (-8.4891, 107.5669) knots 0 0 0 1 2 2 2
  spline S185 degree 2 poles (-8.4891, 107.5669) (-9.3896, 107.5669) (-11.3888, 106.4323) (-12.3254, 105.5498) knots 0 0 0 1 2 2 2
  line L126 (-12.3254, 105.5498) -> (-12.3254, 93.0865)
  line L127 (-12.3254, 93.0865) -> (-15.135, 93.0865)
  line L128 (-15.135, 93.0865) -> (-15.135, 109.7642)
  line L129 (-15.135, 109.7642) -> (-12.3254, 109.7642)
  line L130 (-12.3254, 109.7642) -> (-12.3254, 107.9271)
  spline S186 degree 2 poles (-12.3254, 107.9271) (-11.2267, 109.0258) (-9.0654, 110.2325) (-7.7687, 110.2325) knots 0 0 0 1 2 2 2
  spline S187 degree 2 poles (-7.7687, 110.2325) (-6.2918, 110.2325) (-4.0045, 108.8817) (-3.4101, 107.3508) knots 0 0 0 1 2 2 2
  spline S188 degree 2 poles (-3.4101, 107.3508) (-2.1314, 108.7736) (0.282, 110.2325) (1.6868, 110.2325) knots 0 0 0 1 2 2 2
  spline S189 degree 2 poles (1.6868, 110.2325) (2.7675, 110.2325) (4.5325, 109.5661) (5.1809, 108.8097) knots 0 0 0 1 2 2 2
  spline S190 degree 2 poles (5.1809, 108.8097) (5.8473, 108.0532) (6.5857, 105.7839) (6.5857, 104.0729) knots 0 0 0 1 2 2 2
  line L131 (6.5857, 104.0729) -> (6.5857, 93.0865)
  line L132 (6.5857, 93.0865) -> (3.7761, 93.0865)
  line L133 (13.3937, 93.0865) -> (10.584, 93.0865)
  line L134 (10.584, 93.0865) -> (10.584, 109.7642)
  line L135 (10.584, 109.7642) -> (13.3937, 109.7642)
  line L136 (13.3937, 109.7642) -> (13.3937, 93.0865)
  line L137 (13.5918, 112.5378) -> (10.4039, 112.5378)
  line L138 (10.4039, 112.5378) -> (10.4039, 115.4555)
  line L139 (10.4039, 115.4555) -> (13.5918, 115.4555)
  line L140 (13.5918, 115.4555) -> (13.5918, 112.5378)
  line L141 (30.6118, 93.0865) -> (27.8021, 93.0865)
  line L142 (27.8021, 93.0865) -> (27.8021, 102.596)
  spline S191 degree 2 poles (27.8021, 102.596) (27.8021, 103.7487) (27.586, 105.7299) (27.2618, 106.3242) knots 0 0 0 1 2 2 2
  spline S192 degree 2 poles (27.2618, 106.3242) (26.9196, 106.9546) (25.6949, 107.5669) (24.6503, 107.5669) knots 0 0 0 1 2 2 2
  spline S193 degree 2 poles (24.6503, 107.5669) (23.6057, 107.5669) (21.3904, 106.4503) (20.3277, 105.5498) knots 0 0 0 1 2 2 2
  line L143 (20.3277, 105.5498) -> (20.3277, 93.0865)
  line L144 (20.3277, 93.0865) -> (17.5181, 93.0865)
  line L145 (17.5181, 93.0865) -> (17.5181, 109.7642)
  line L146 (17.5181, 109.7642) -> (20.3277, 109.7642)
  line L147 (20.3277, 109.7642) -> (20.3277, 107.9091)
  spline S194 degree 2 poles (20.3277, 107.9091) (21.5885, 109.0438) (24.0199, 110.2325) (25.3887, 110.2325) knots 0 0 0 1 2 2 2
  spline S195 degree 2 poles (25.3887, 110.2325) (27.8381, 110.2325) (30.6118, 106.9906) (30.6118, 103.9108) knots 0 0 0 1 2 2 2
  line L148 (30.6118, 103.9108) -> (30.6118, 93.0865)
  line L149 (47.5237, 93.0865) -> (44.714, 93.0865)
  line L150 (44.714, 93.0865) -> (44.714, 94.9235)
  spline S196 degree 2 poles (44.714, 94.9235) (43.4173, 93.7889) (41.0939, 92.6182) (39.6531, 92.6182) knots 0 0 0 1 2 2 2
  spline S197 degree 2 poles (39.6531, 92.6182) (38.5724, 92.6182) (36.6453, 93.3386) (35.9429, 94.1131) knots 0 0 0 1 2 2 2
  spline S198 degree 2 poles (35.9429, 94.1131) (35.2225, 94.8875) (34.43, 97.2469) (34.43, 98.9399) knots 0 0 0 1 2 2 2
  line L151 (34.43, 98.9399) -> (34.43, 109.7642)
  line L152 (34.43, 109.7642) -> (37.2396, 109.7642)
  line L153 (37.2396, 109.7642) -> (37.2396, 100.2547)
  spline S199 degree 2 poles (37.2396, 100.2547) (37.2396, 98.9219) (37.4378, 97.1749) (37.78, 96.5265) knots 0 0 0 1 2 2 2
  spline S200 degree 2 poles (37.78, 96.5265) (38.1222, 95.8781) (39.2928, 95.2837) (40.3915, 95.2837) knots 0 0 0 1 2 2 2
  spline S201 degree 2 poles (40.3915, 95.2837) (41.4181, 95.2837) (43.7414, 96.4544) (44.714, 97.3009) knots 0 0 0 1 2 2 2
  line L154 (44.714, 97.3009) -> (44.714, 109.7642)
  line L155 (44.714, 109.7642) -> (47.5237, 109.7642)
  line L156 (47.5237, 109.7642) -> (47.5237, 93.0865)
  spline S202 degree 2 poles (56.637, 92.7623) (54.3497, 92.7623) (51.7741, 95.3738) (51.7741, 98.2015) knots 0 0 0 1 2 2 2
  line L157 (51.7741, 98.2015) -> (51.7741, 107.4409)
  line L158 (51.7741, 107.4409) -> (49.883, 107.4409)
  line L159 (49.883, 107.4409) -> (49.883, 109.7642)
  line L160 (49.883, 109.7642) -> (51.7741, 109.7642)
  line L161 (51.7741, 109.7642) -> (51.7741, 114.555)
  line L162 (51.7741, 114.555) -> (54.5838, 114.555)
  line L163 (54.5838, 114.555) -> (54.5838, 109.7642)
  line L164 (54.5838, 109.7642) -> (59.7528, 109.7642)
  line L165 (59.7528, 109.7642) -> (59.7528, 107.4409)
  line L166 (59.7528, 107.4409) -> (54.5838, 107.4409)
  line L167 (54.5838, 107.4409) -> (54.5838, 99.4982)
  spline S203 degree 2 poles (54.5838, 99.4982) (54.5838, 98.2375) (54.6738, 96.8507) (54.98, 96.2563) knots 0 0 0 1 2 2 2
  spline S204 degree 2 poles (54.98, 96.2563) (55.2322, 95.734) (56.3668, 95.2117) (57.3394, 95.2117) knots 0 0 0 1 2 2 2
  spline S205 degree 2 poles (57.3394, 95.2117) (58.0238, 95.2117) (59.3025, 95.6259) (59.5907, 95.752) knots 0 0 0 1 2 2 2
  line L168 (59.5907, 95.752) -> (59.7528, 95.752)
  line L169 (59.7528, 95.752) -> (59.7528, 93.2305)
  spline S206 degree 2 poles (59.7528, 93.2305) (58.9603, 93.0144) (57.3394, 92.7623) (56.637, 92.7623) knots 0 0 0 1 2 2 2
  spline S207 degree 2 poles (69.0643, 92.7082) (65.0659, 92.7082) (60.6713, 97.1929) (60.6713, 101.3353) knots 0 0 0 1 2 2 2
  spline S208 degree 2 poles (60.6713, 101.3353) (60.6713, 105.4057) (64.9398, 110.2325) (68.3799, 110.2325) knots 0 0 0 1 2 2 2
  spline S209 degree 2 poles (68.3799, 110.2325) (69.9288, 110.2325) (72.3242, 109.332) (73.2067, 108.3774) knots 0 0 0 1 2 2 2
  spline S210 degree 2 poles (73.2067, 108.3774) (74.1072, 107.4229) (75.0618, 104.6672) (75.0618, 102.6681) knots 0 0 0 1 2 2 2
  line L170 (75.0618, 102.6681) -> (75.0618, 101.1372)
  line L171 (75.0618, 101.1372) -> (63.517, 101.1372)
  spline S211 degree 2 poles (63.517, 101.1372) (63.517, 98.2375) (66.4347, 95.1577) (69.0282, 95.1577) knots 0 0 0 1 2 2 2
  spline S212 degree 2 poles (69.0282, 95.1577) (69.9468, 95.1577) (71.7298, 95.5719) (72.4502, 95.8961) knots 0 0 0 1 2 2 2
  spline S213 degree 2 poles (72.4502, 95.8961) (73.2067, 96.2563) (74.2513, 96.8867) (74.5935, 97.1749) knots 0 0 0 1 2 2 2
  line L172 (74.5935, 97.1749) -> (74.7556, 97.1749)
  line L173 (74.7556, 97.1749) -> (74.7556, 94.1131)
  spline S214 degree 2 poles (74.7556, 94.1131) (74.2693, 93.9149) (72.7924, 93.3386) (72.2161, 93.1765) knots 0 0 0 1 2 2 2
  spline S215 degree 2 poles (72.2161, 93.1765) (71.4056, 92.9424) (70.0728, 92.7082) (69.0643, 92.7082) knots 0 0 0 1 2 2 2
  spline S216 degree 2 poles (72.3242, 103.2804) (72.2881, 104.4151) (71.8199, 106.0721) (71.3696, 106.6304) knots 0 0 0 1 2 2 2
  spline S217 degree 2 poles (71.3696, 106.6304) (70.8833, 107.2608) (69.3524, 107.9271) (68.2178, 107.9271) knots 0 0 0 1 2 2 2
  spline S218 degree 2 poles (68.2178, 107.9271) (67.1011, 107.9271) (65.5342, 107.2608) (64.8858, 106.6124) knots 0 0 0 1 2 2 2
  spline S219 degree 2 poles (64.8858, 106.6124) (64.2554, 105.946) (63.6071, 104.343) (63.517, 103.2804) knots 0 0 0 1 2 2 2
  line L174 (63.517, 103.2804) -> (72.3242, 103.2804)
  spline S220 degree 2 poles (-20.5021, 57.4836) (-20.8443, 57.2315) (-21.997, 56.331) (-22.5373, 56.0608) knots 0 0 0 1 2 2 2
  spline S221 degree 2 poles (-22.5373, 56.0608) (-23.2758, 55.6646) (-24.6626, 55.2503) (-25.9233, 55.2503) knots 0 0 0 1 2 2 2
  spline S222 degree 2 poles (-25.9233, 55.2503) (-26.9499, 55.2503) (-28.805, 56.0248) (-29.5074, 56.7272) knots 0 0 0 1 2 2 2
  spline S223 degree 2 poles (-29.5074, 56.7272) (-30.1738, 57.4116) (-30.9843, 59.4288) (-30.9843, 60.5454) knots 0 0 0 1 2 2 2
  spline S224 degree 2 poles (-30.9843, 60.5454) (-30.9843, 62.2744) (-29.5254, 64.7239) (-27.9405, 65.4263) knots 0 0 0 1 2 2 2
  spline S225 degree 2 poles (-27.9405, 65.4263) (-26.5357, 66.0747) (-22.7174, 66.561) (-20.5021, 66.687) knots 0 0 0 1 2 2 2
  line L175 (-20.5021, 66.687) -> (-20.5021, 67.2273)
  spline S226 degree 2 poles (-20.5021, 67.2273) (-20.5021, 68.1999) (-21.0965, 69.4066) (-21.6368, 69.7488) knots 0 0 0 1 2 2 2
  spline S227 degree 2 poles (-21.6368, 69.7488) (-22.1771, 70.091) (-23.726, 70.3071) (-24.5545, 70.3071) knots 0 0 0 1 2 2 2
  spline S228 degree 2 poles (-24.5545, 70.3071) (-25.5271, 70.3071) (-28.1566, 69.7308) (-29.4714, 69.1725) knots 0 0 0 1 2 2 2
  line L176 (-29.4714, 69.1725) -> (-29.6335, 69.1725)
  line L177 (-29.6335, 69.1725) -> (-29.6335, 72.0362)
  spline S229 degree 2 poles (-29.6335, 72.0362) (-28.859, 72.2523) (-25.9593, 72.7926) (-24.5365, 72.7926) knots 0 0 0 1 2 2 2
  spline S230 degree 2 poles (-24.5365, 72.7926) (-22.8075, 72.7926) (-20.4481, 72.2523) (-19.5116, 71.5499) knots 0 0 0 1 2 2 2
  spline S231 degree 2 poles (-19.5116, 71.5499) (-18.593, 70.8655) (-17.6925, 68.6862) (-17.6925, 67.1193) knots 0 0 0 1 2 2 2
  line L178 (-17.6925, 67.1193) -> (-17.6925, 55.7186)
  line L179 (-17.6925, 55.7186) -> (-20.5021, 55.7186)
  line L180 (-20.5021, 55.7186) -> (-20.5021, 57.4836)
  line L181 (-20.5021, 59.825) -> (-20.5021, 64.4537)
  spline S232 degree 2 poles (-20.5021, 64.4537) (-21.5107, 64.3637) (-24.5545, 64.0575) (-25.5091, 63.7693) knots 0 0 0 1 2 2 2
  spline S233 degree 2 poles (-25.5091, 63.7693) (-26.6257, 63.4271) (-28.0846, 62.0043) (-28.0846, 60.7436) knots 0 0 0 1 2 2 2
  spline S234 degree 2 poles (-28.0846, 60.7436) (-28.0846, 59.3027) (-26.4636, 57.8439) (-24.9147, 57.8439) knots 0 0 0 1 2 2 2
  spline S235 degree 2 poles (-24.9147, 57.8439) (-23.5999, 57.8439) (-21.4387, 58.9785) (-20.5021, 59.825) knots 0 0 0 1 2 2 2
  line L182 (-4.9771, 76.2326) -> (-5.1211, 76.2326)
  spline S236 degree 2 poles (-5.1211, 76.2326) (-5.4994, 76.3767) (-6.9042, 76.6288) (-7.4625, 76.6288) knots 0 0 0 1 2 2 2
  spline S237 degree 2 poles (-7.4625, 76.6288) (-9.2275, 76.6288) (-10.7404, 75.0439) (-10.7404, 72.9547) knots 0 0 0 1 2 2 2
  line L183 (-10.7404, 72.9547) -> (-10.7404, 72.3964)
  line L184 (-10.7404, 72.3964) -> (-6.0937, 72.3964)
  line L185 (-6.0937, 72.3964) -> (-6.0937, 70.073)
  line L186 (-6.0937, 70.073) -> (-10.6504, 70.073)
  line L187 (-10.6504, 70.073) -> (-10.6504, 55.7186)
  line L188 (-10.6504, 55.7186) -> (-13.46, 55.7186)
  line L189 (-13.46, 55.7186) -> (-13.46, 70.073)
  line L190 (-13.46, 70.073) -> (-15.3511, 70.073)
  line L191 (-15.3511, 70.073) -> (-15.3511, 72.3964)
  line L192 (-15.3511, 72.3964) -> (-13.46, 72.3964)
  line L193 (-13.46, 72.3964) -> (-13.46, 72.9547)
  spline S238 degree 2 poles (-13.46, 72.9547) (-13.46, 75.9444) (-10.5603, 79.0783) (-7.8587, 79.0783) knots 0 0 0 1 2 2 2
  spline S239 degree 2 poles (-7.8587, 79.0783) (-7.0843, 79.0783) (-5.5894, 78.9162) (-4.9771, 78.8081) knots 0 0 0 1 2 2 2
  line L194 (-4.9771, 78.8081) -> (-4.9771, 76.2326)
  spline S240 degree 2 poles (1.6688, 55.3944) (-0.6185, 55.3944) (-3.194, 58.006) (-3.194, 60.8336) knots 0 0 0 1 2 2 2
  line L195 (-3.194, 60.8336) -> (-3.194, 70.073)
  line L196 (-3.194, 70.073) -> (-5.0851, 70.073)
  line L197 (-5.0851, 70.073) -> (-5.0851, 72.3964)
  line L198 (-5.0851, 72.3964) -> (-3.194, 72.3964)
  line L199 (-3.194, 72.3964) -> (-3.194, 77.1872)
  line L200 (-3.194, 77.1872) -> (-0.3844, 77.1872)
  line L201 (-0.3844, 77.1872) -> (-0.3844, 72.3964)
  line L202 (-0.3844, 72.3964) -> (4.7847, 72.3964)
  line L203 (4.7847, 72.3964) -> (4.7847, 70.073)
  line L204 (4.7847, 70.073) -> (-0.3844, 70.073)
  line L205 (-0.3844, 70.073) -> (-0.3844, 62.1304)
  spline S241 degree 2 poles (-0.3844, 62.1304) (-0.3844, 60.8696) (-0.2943, 59.4828) (0.0119, 58.8885) knots 0 0 0 1 2 2 2
  spline S242 degree 2 poles (0.0119, 58.8885) (0.264, 58.3662) (1.3987, 57.8439) (2.3712, 57.8439) knots 0 0 0 1 2 2 2
  spline S243 degree 2 poles (2.3712, 57.8439) (3.0556, 57.8439) (4.3344, 58.2581) (4.6226, 58.3842) knots 0 0 0 1 2 2 2
  line L206 (4.6226, 58.3842) -> (4.7847, 58.3842)
  line L207 (4.7847, 58.3842) -> (4.7847, 55.8627)
  spline S244 degree 2 poles (4.7847, 55.8627) (3.9922, 55.6466) (2.3712, 55.3944) (1.6688, 55.3944) knots 0 0 0 1 2 2 2
  spline S245 degree 2 poles (14.0961, 55.3404) (10.0978, 55.3404) (5.7032, 59.825) (5.7032, 63.9674) knots 0 0 0 1 2 2 2
  spline S246 degree 2 poles (5.7032, 63.9674) (5.7032, 68.0378) (9.9717, 72.8646) (13.4117, 72.8646) knots 0 0 0 1 2 2 2
  spline S247 degree 2 poles (13.4117, 72.8646) (14.9606, 72.8646) (17.356, 71.9641) (18.2385, 71.0096) knots 0 0 0 1 2 2 2
  spline S248 degree 2 poles (18.2385, 71.0096) (19.1391, 70.055) (20.0936, 67.2994) (20.0936, 65.3002) knots 0 0 0 1 2 2 2
  line L208 (20.0936, 65.3002) -> (20.0936, 63.7693)
  line L209 (20.0936, 63.7693) -> (8.5489, 63.7693)
  spline S249 degree 2 poles (8.5489, 63.7693) (8.5489, 60.8696) (11.4666, 57.7898) (14.0601, 57.7898) knots 0 0 0 1 2 2 2
  spline S250 degree 2 poles (14.0601, 57.7898) (14.9786, 57.7898) (16.7617, 58.2041) (17.4821, 58.5283) knots 0 0 0 1 2 2 2
  spline S251 degree 2 poles (17.4821, 58.5283) (18.2385, 58.8885) (19.2831, 59.5188) (19.6253, 59.807) knots 0 0 0 1 2 2 2
  line L210 (19.6253, 59.807) -> (19.7874, 59.807)
  line L211 (19.7874, 59.807) -> (19.7874, 56.7452)
  spline S252 degree 2 poles (19.7874, 56.7452) (19.3011, 56.5471) (17.8243, 55.9708) (17.2479, 55.8087) knots 0 0 0 1 2 2 2
  spline S253 degree 2 poles (17.2479, 55.8087) (16.4375, 55.5745) (15.1047, 55.3404) (14.0961, 55.3404) knots 0 0 0 1 2 2 2
  spline S254 degree 2 poles (17.356, 65.9126) (17.32, 67.0472) (16.8517, 68.7042) (16.4015, 69.2625) knots 0 0 0 1 2 2 2
  spline S255 degree 2 poles (16.4015, 69.2625) (15.9152, 69.8929) (14.3843, 70.5593) (13.2496, 70.5593) knots 0 0 0 1 2 2 2
  spline S256 degree 2 poles (13.2496, 70.5593) (12.133, 70.5593) (10.566, 69.8929) (9.9177, 69.2445) knots 0 0 0 1 2 2 2
  spline S257 degree 2 poles (9.9177, 69.2445) (9.2873, 68.5781) (8.6389, 66.9752) (8.5489, 65.9126) knots 0 0 0 1 2 2 2
  line L212 (8.5489, 65.9126) -> (17.356, 65.9126)
  line L213 (31.7824, 69.3886) -> (31.6384, 69.3886)
  spline S258 degree 2 poles (31.6384, 69.3886) (31.3142, 69.4787) (30.6118, 69.5147) (30.1255, 69.5147) knots 0 0 0 1 2 2 2
  spline S259 degree 2 poles (30.1255, 69.5147) (28.9908, 69.5147) (26.7575, 68.5241) (25.7489, 67.5515) knots 0 0 0 1 2 2 2
  line L214 (25.7489, 67.5515) -> (25.7489, 55.7186)
  line L215 (25.7489, 55.7186) -> (22.9393, 55.7186)
  line L216 (22.9393, 55.7186) -> (22.9393, 72.3964)
  line L217 (22.9393, 72.3964) -> (25.7489, 72.3964)
  line L218 (25.7489, 72.3964) -> (25.7489, 69.9109)
  spline S260 degree 2 poles (25.7489, 69.9109) (27.2798, 71.2797) (29.5672, 72.3964) (30.6478, 72.3964) knots 0 0 0 1 2 2 2
  spline S261 degree 2 poles (30.6478, 72.3964) (31.08, 72.3964) (31.5123, 72.3603) (31.7824, 72.3063) knots 0 0 0 1 2 2 2
  line L219 (31.7824, 72.3063) -> (31.7824, 69.3886)
  spline S262 degree 2 poles (-38.2965, 27.6802) (-38.2965, 23.4658) (-42.3489, 18.8731) (-45.7349, 18.8731) knots 0 0 0 1 2 2 2
  spline S263 degree 2 poles (-45.7349, 18.8731) (-49.2109, 18.8731) (-53.1913, 23.6098) (-53.1913, 27.6802) knots 0 0 0 1 2 2 2
  spline S264 degree 2 poles (-53.1913, 27.6802) (-53.1913, 31.8587) (-49.0849, 36.4874) (-45.7349, 36.4874) knots 0 0 0 1 2 2 2
  spline S265 degree 2 poles (-45.7349, 36.4874) (-42.3489, 36.4874) (-38.2965, 31.8767) (-38.2965, 27.6802) knots 0 0 0 1 2 2 2
  spline S266 degree 2 poles (-41.1962, 27.6802) (-41.1962, 30.9221) (-43.5556, 34.074) (-45.7349, 34.074) knots 0 0 0 1 2 2 2
  spline S267 degree 2 poles (-45.7349, 34.074) (-47.9142, 34.074) (-50.2916, 30.9221) (-50.2916, 27.6802) knots 0 0 0 1 2 2 2
  spline S268 degree 2 poles (-50.2916, 27.6802) (-50.2916, 24.5284) (-47.9142, 21.2865) (-45.7349, 21.2865) knots 0 0 0 1 2 2 2
  spline S269 degree 2 poles (-45.7349, 21.2865) (-43.5736, 21.2865) (-41.1962, 24.4743) (-41.1962, 27.6802) knots 0 0 0 1 2 2 2
  spline S270 degree 2 poles (-21.4387, 28.1305) (-21.4387, 23.952) (-25.419, 19.0172) (-28.4628, 19.0172) knots 0 0 0 1 2 2 2
  spline S271 degree 2 poles (-28.4628, 19.0172) (-29.7055, 19.0172) (-31.6146, 19.5935) (-32.6052, 20.1878) knots 0 0 0 1 2 2 2
  line L220 (-32.6052, 20.1878) -> (-32.6052, 13.1998)
  line L221 (-32.6052, 13.1998) -> (-35.4149, 13.1998)
  line L222 (-35.4149, 13.1998) -> (-35.4149, 36.0191)
  line L223 (-35.4149, 36.0191) -> (-32.6052, 36.0191)
  line L224 (-32.6052, 36.0191) -> (-32.6052, 34.2721)
  spline S272 degree 2 poles (-32.6052, 34.2721) (-31.5606, 35.2266) (-29.0031, 36.4874) (-27.5082, 36.4874) knots 0 0 0 1 2 2 2
  spline S273 degree 2 poles (-27.5082, 36.4874) (-24.6446, 36.4874) (-21.4387, 31.9487) (-21.4387, 28.1305) knots 0 0 0 1 2 2 2
  spline S274 degree 2 poles (-24.3384, 27.8063) (-24.3384, 30.67) (-26.1574, 33.8218) (-28.1926, 33.8218) knots 0 0 0 1 2 2 2
  spline S275 degree 2 poles (-28.1926, 33.8218) (-29.3813, 33.8218) (-31.6146, 32.7592) (-32.6052, 31.9307) knots 0 0 0 1 2 2 2
  line L225 (-32.6052, 31.9307) -> (-32.6052, 22.4572)
  spline S276 degree 2 poles (-32.6052, 22.4572) (-31.5066, 21.9349) (-29.9397, 21.5386) (-28.9311, 21.5386) knots 0 0 0 1 2 2 2
  spline S277 degree 2 poles (-28.9311, 21.5386) (-26.7518, 21.5386) (-24.3384, 24.7445) (-24.3384, 27.8063) knots 0 0 0 1 2 2 2
  spline S278 degree 2 poles (-11.2807, 18.9631) (-15.2791, 18.9631) (-19.6737, 23.4477) (-19.6737, 27.5902) knots 0 0 0 1 2 2 2
  spline S279 degree 2 poles (-19.6737, 27.5902) (-19.6737, 31.6606) (-15.4052, 36.4874) (-11.9651, 36.4874) knots 0 0 0 1 2 2 2